Autodesk Fusion 360 part; units mm, degrees
note: some values were not read from the file. Chosen so that the rebuilt part matches the saved one: which face or edge a step refers to. Set by a fixed rule: which sketch regions a step uses.
(part 5 of 7)
  arc A238 (-20.6449, 76.0422) -> (-22.1292, 75.6235) centre (0, 0) ccw
  arc A239 (-20.6449, 76.0422) -> (-20.3501, 76.41) centre (-20.7497, 76.4282) ccw
  spline S239 degree 3 poles (-20.3133, 77.0419) (-20.3288, 76.8232) (-20.341, 76.6126) (-20.3501, 76.41) knots 0 0 0 0 1 1 1 1
  spline S240 degree 3 poles (-19.9812, 79.7947) (-20.1522, 78.771) (-20.2559, 77.8517) (-20.3133, 77.0419) knots 0 0 0 0 1 1 1 1
  arc A240 (-18.4227, 80.1689) -> (-19.9812, 79.7947) centre (0, 0) ccw
  spline S241 degree 3 poles (-16.877, 77.8669) (-17.2958, 78.5624) (-17.8055, 79.3344) (-18.4227, 80.1689) knots 0 0 0 0 1 1 1 1
  spline S242 degree 3 poles (-16.5573, 77.3206) (-16.6574, 77.4969) (-16.7639, 77.6791) (-16.877, 77.8669) knots 0 0 0 0 1 1 1 1
  arc A241 (-16.5573, 77.3206) -> (-16.1277, 77.1267) centre (-16.2095, 77.5182) ccw
  arc A242 (-14.6151, 77.4275) -> (-16.1277, 77.1267) centre (0, 0) ccw
  arc A243 (-14.6151, 77.4275) -> (-14.2923, 77.7712) centre (-14.6893, 77.8206) ccw
  spline S243 degree 3 poles (-14.2061, 78.3982) (-14.2387, 78.1814) (-14.2673, 77.9723) (-14.2923, 77.7712) knots 0 0 0 0 1 1 1 1
  spline S244 degree 3 poles (-13.659, 81.1164) (-13.9098, 80.1093) (-14.0853, 79.201) (-14.2061, 78.3982) knots 0 0 0 0 1 1 1 1
  arc A244 (-12.0759, 81.3672) -> (-13.659, 81.1164) centre (0, 0) ccw
  spline S245 degree 3 poles (-10.7156, 78.951) (-11.0785, 79.6772) (-11.5261, 80.4868) (-12.0759, 81.3672) knots 0 0 0 0 1 1 1 1
  spline S246 degree 3 poles (-10.4398, 78.3813) (-10.5258, 78.5649) (-10.6176, 78.7549) (-10.7156, 78.951) knots 0 0 0 0 1 1 1 1
  arc A245 (-10.4398, 78.3813) -> (-10.0267, 78.1543) centre (-10.0776, 78.551) ccw
  arc A246 (-8.4951, 78.3355) -> (-10.0267, 78.1543) centre (0, 0) ccw
  arc A247 (-8.4951, 78.3355) -> (-8.1464, 78.6528) centre (-8.5383, 78.7332) ccw
  spline S247 degree 3 poles (-8.0112, 79.2711) (-8.0608, 79.0575) (-8.1057, 78.8514) (-8.1464, 78.6528) knots 0 0 0 0 1 1 1 1
  spline S248 degree 3 poles (-7.2526, 81.938) (-7.5816, 80.9537) (-7.8278, 80.0619) (-8.0112, 79.2711) knots 0 0 0 0 1 1 1 1
  arc A248 (-5.6547, 82.0638) -> (-7.2526, 81.938) centre (0, 0) ccw
  spline S249 degree 3 poles (-4.4881, 79.5484) (-4.793, 80.3008) (-5.1757, 81.1431) (-5.6547, 82.0638) knots 0 0 0 0 1 1 1 1
  spline S250 degree 3 poles (-4.2579, 78.9588) (-4.3292, 79.1486) (-4.4058, 79.3452) (-4.4881, 79.5484) knots 0 0 0 0 1 1 1 1
  arc A249 (-4.2579, 78.9588) -> (-3.8638, 78.7) centre (-3.8835, 79.0995) ccw
  arc A250 (-2.3228, 78.7606) -> (-3.8638, 78.7) centre (0, 0) ccw
  arc A251 (-2.3228, 78.7606) -> (-1.9503, 79.0495) centre (-2.3346, 79.1604) ccw
  spline S251 degree 3 poles (-1.767, 79.6553) (-1.8331, 79.4462) (-1.8941, 79.2443) (-1.9503, 79.0495) knots 0 0 0 0 1 1 1 1
  spline S252 degree 3 poles (-0.8014, 82.2545) (-1.2067, 81.299) (-1.5221, 80.4293) (-1.767, 79.6553) knots 0 0 0 0 1 1 1 1
  arc A252 (0.8014, 82.2545) -> (-0.8014, 82.2545) centre (0, 0) ccw
  spline S253 degree 3 poles (1.767, 79.6553) (1.5221, 80.4293) (1.2067, 81.299) (0.8014, 82.2545) knots 0 0 0 0 1 1 1 1
  spline S254 degree 3 poles (1.9503, 79.0495) (1.8941, 79.2443) (1.8331, 79.4462) (1.767, 79.6553) knots 0 0 0 0 1 1 1 1
  arc A253 (1.9503, 79.0495) -> (2.3228, 78.7606) centre (2.3346, 79.1604) ccw
  arc A254 (3.8638, 78.7) -> (2.3228, 78.7606) centre (0, 0) ccw
  arc A255 (3.8638, 78.7) -> (4.2579, 78.9588) centre (3.8835, 79.0995) ccw
  spline S255 degree 3 poles (4.4881, 79.5484) (4.4058, 79.3452) (4.3292, 79.1486) (4.2579, 78.9588) knots 0 0 0 0 1 1 1 1
  spline S256 degree 3 poles (5.6547, 82.0638) (5.1757, 81.1431) (4.793, 80.3008) (4.4881, 79.5484) knots 0 0 0 0 1 1 1 1
  arc A256 (7.2526, 81.938) -> (5.6547, 82.0638) centre (0, 0) ccw
  spline S257 degree 3 poles (8.0112, 79.2711) (7.8278, 80.0619) (7.5816, 80.9537) (7.2526, 81.938) knots 0 0 0 0 1 1 1 1
  spline S258 degree 3 poles (8.1464, 78.6528) (8.1057, 78.8514) (8.0608, 79.0575) (8.0112, 79.2711) knots 0 0 0 0 1 1 1 1
  arc A257 (8.1464, 78.6528) -> (8.4951, 78.3355) centre (8.5383, 78.7332) ccw
  arc A258 (10.0267, 78.1543) -> (8.4951, 78.3355) centre (0, 0) ccw
  arc A259 (10.0267, 78.1543) -> (10.4398, 78.3813) centre (10.0776, 78.551) ccw
  spline S259 degree 3 poles (10.7156, 78.951) (10.6176, 78.7549) (10.5258, 78.5649) (10.4398, 78.3813) knots 0 0 0 0 1 1 1 1
  spline S260 degree 3 poles (12.0759, 81.3672) (11.5261, 80.4868) (11.0785, 79.6772) (10.7156, 78.951) knots 0 0 0 0 1 1 1 1
  arc A260 (13.659, 81.1164) -> (12.0759, 81.3672) centre (0, 0) ccw
  spline S261 degree 3 poles (14.2061, 78.3982) (14.0853, 79.201) (13.9098, 80.1093) (13.659, 81.1164) knots 0 0 0 0 1 1 1 1
  spline S262 degree 3 poles (14.2923, 77.7712) (14.2673, 77.9723) (14.2387, 78.1814) (14.2061, 78.3982) knots 0 0 0 0 1 1 1 1
  arc A261 (14.2923, 77.7712) -> (14.6151, 77.4275) centre (14.6893, 77.8206) ccw
  arc A262 (16.1277, 77.1267) -> (14.6151, 77.4275) centre (0, 0) ccw
  arc A263 (16.1277, 77.1267) -> (16.5573, 77.3206) centre (16.2095, 77.5182) ccw
  spline S263 degree 3 poles (16.877, 77.8669) (16.7639, 77.6791) (16.6574, 77.4969) (16.5573, 77.3206) knots 0 0 0 0 1 1 1 1
  spline S264 degree 3 poles (18.4227, 80.1689) (17.8055, 79.3344) (17.2958, 78.5624) (16.877, 77.8669) knots 0 0 0 0 1 1 1 1
  arc A264 (19.9812, 79.7947) -> (18.4227, 80.1689) centre (0, 0) ccw
  spline S265 degree 3 poles (20.3133, 77.0419) (20.2559, 77.8517) (20.1522, 78.771) (19.9812, 79.7947) knots 0 0 0 0 1 1 1 1
  spline S266 degree 3 poles (20.3501, 76.41) (20.341, 76.6126) (20.3288, 76.8232) (20.3133, 77.0419) knots 0 0 0 0 1 1 1 1
  arc A265 (20.3501, 76.41) -> (20.6449, 76.0422) centre (20.7497, 76.4282) ccw
  arc A266 (22.1292, 75.6235) -> (20.6449, 76.0422) centre (0, 0) ccw
  arc A267 (22.1292, 75.6235) -> (22.5728, 75.7832) centre (22.2416, 76.0074) ccw
  spline S267 degree 3 poles (22.9343, 76.3027) (22.8068, 76.1243) (22.6864, 75.9511) (22.5728, 75.7832) knots 0 0 0 0 1 1 1 1
  spline S268 degree 3 poles (24.6558, 78.4763) (23.9752, 77.6928) (23.4064, 76.9632) (22.9343, 76.3027) knots 0 0 0 0 1 1 1 1
  arc A268 (26.1802, 77.981) -> (24.6558, 78.4763) centre (0, 0) ccw
  spline S269 degree 3 poles (26.2953, 75.2107) (26.3016, 76.0225) (26.2704, 76.9471) (26.1802, 77.981) knots 0 0 0 0 1 1 1 1
  spline S270 degree 3 poles (26.2825, 74.5778) (26.2892, 74.7805) (26.2937, 74.9914) (26.2953, 75.2107) knots 0 0 0 0 1 1 1 1
  arc A269 (26.2825, 74.5778) -> (26.5475, 74.188) centre (26.6822, 74.5646) ccw
  arc A270 (27.9944, 73.6542) -> (26.5475, 74.188) centre (0, 0) ccw
  arc A271 (27.9944, 73.6542) -> (28.4491, 73.7785) centre (28.1365, 74.0281) ccw
  spline S271 degree 3 poles (28.8503, 74.2681) (28.7092, 74.1003) (28.5755, 73.937) (28.4491, 73.7785) knots 0 0 0 0 1 1 1 1
  spline S272 degree 3 poles (30.737, 76.2999) (29.997, 75.5723) (29.3727, 74.8895) (28.8503, 74.2681) knots 0 0 0 0 1 1 1 1
  arc A272 (32.2178, 75.6865) -> (30.737, 76.2999) centre (0, 0) ccw
  spline S273 degree 3 poles (32.1152, 72.9157) (32.1852, 73.7245) (32.2266, 74.6487) (32.2178, 75.6865) knots 0 0 0 0 1 1 1 1
  spline S274 degree 3 poles (32.0528, 72.2858) (32.0754, 72.4873) (32.0964, 72.6972) (32.1152, 72.9157) knots 0 0 0 0 1 1 1 1
  arc A273 (32.0528, 72.2858) -> (32.2864, 71.8764) centre (32.4503, 72.2413) ccw
  arc A274 (33.6869, 71.2307) -> (32.2864, 71.8764) centre (0, 0) ccw
  arc A275 (33.6869, 71.2307) -> (34.15, 71.319) centre (33.8579, 71.5923) ccw
  spline S275 degree 3 poles (34.5883, 71.7756) (34.4345, 71.6193) (34.2885, 71.4671) (34.15, 71.319) knots 0 0 0 0 1 1 1 1
  spline S276 degree 3 poles (36.6287, 73.6531) (35.8338, 72.9858) (35.1579, 72.3541) (34.5883, 71.7756) knots 0 0 0 0 1 1 1 1
  arc A276 (38.0568, 72.9254) -> (36.6287, 73.6531) centre (0, 0) ccw
  spline S277 degree 3 poles (37.7371, 70.1712) (37.8704, 70.972) (37.9841, 71.8901) (38.0568, 72.9254) knots 0 0 0 0 1 1 1 1
  spline S278 degree 3 poles (37.6254, 69.5482) (37.6638, 69.7473) (37.7012, 69.9549) (37.7371, 70.1712) knots 0 0 0 0 1 1 1 1
  arc A277 (37.6254, 69.5482) -> (37.8262, 69.1217) centre (38.0182, 69.4726) ccw
  arc A278 (39.1718, 68.3681) -> (37.8262, 69.1217) centre (0, 0) ccw
  arc A279 (39.1718, 68.3681) -> (39.6403, 68.4198) centre (39.3706, 68.7152) ccw
  spline S279 degree 3 poles (40.1132, 68.8406) (39.9475, 68.6969) (39.79, 68.5565) (39.6403, 68.4198) knots 0 0 0 0 1 1 1 1
  spline S280 degree 3 poles (42.2945, 70.5522) (41.4498, 69.9493) (40.7264, 69.3726) (40.1132, 68.8406) knots 0 0 0 0 1 1 1 1
  arc A280 (43.6612, 69.7147) -> (42.2945, 70.5522) centre (0, 0) ccw
  spline S281 degree 3 poles (43.1264, 66.9941) (43.322, 67.7819) (43.5075, 68.6883) (43.6612, 69.7147) knots 0 0 0 0 1 1 1 1
  spline S282 degree 3 poles (42.9661, 66.3817) (43.02, 66.5772) (43.0736, 66.7812) (43.1264, 66.9941) knots 0 0 0 0 1 1 1 1
  arc A281 (42.9661, 66.3817) -> (43.1328, 65.9408) centre (43.3518, 66.2755) ccw
  arc A282 (44.4151, 65.084) -> (43.1328, 65.9408) centre (0, 0) ccw
  arc A283 (44.4151, 65.084) -> (44.8863, 65.0987) centre (44.6406, 65.4144) ccw
  spline S283 degree 3 poles (45.3907, 65.4811) (45.2143, 65.3508) (45.0463, 65.2233) (44.8863, 65.0987) knots 0 0 0 0 1 1 1 1
  spline S284 degree 3 poles (47.6996, 67.0163) (46.8101, 66.4815) (46.0437, 65.9633) (45.3907, 65.4811) knots 0 0 0 0 1 1 1 1
  arc A284 (48.9963, 66.0742) -> (47.6996, 67.0163) centre (0, 0) ccw
  spline S285 degree 3 poles (48.2497, 63.4039) (48.5066, 64.174) (48.7626, 65.063) (48.9963, 66.0742) knots 0 0 0 0 1 1 1 1
  spline S286 degree 3 poles (48.0419, 62.806) (48.111, 62.9966) (48.1804, 63.1959) (48.2497, 63.4039) knots 0 0 0 0 1 1 1 1
  arc A285 (48.0419, 62.806) -> (48.1735, 62.3533) centre (48.418, 62.6699) ccw
  arc A286 (49.3846, 61.3986) -> (48.1735, 62.3533) centre (0, 0) ccw
  arc A287 (49.3846, 61.3986) -> (49.8555, 61.3763) centre (49.6353, 61.7102) ccw
  spline S287 degree 3 poles (50.3883, 61.7179) (50.2023, 61.6019) (50.0247, 61.4879) (49.8555, 61.3763) knots 0 0 0 0 1 1 1 1
  spline S288 degree 3 poles (52.8106, 63.0673) (51.8819, 62.6039) (51.0772, 62.1475) (50.3883, 61.7179) knots 0 0 0 0 1 1 1 1
  arc A288 (54.0294, 62.0263) -> (52.8106, 63.0673) centre (0, 0) ccw
  spline S289 degree 3 poles (53.0756, 59.4228) (53.3921, 60.1704) (53.717, 61.0366) (54.0294, 62.0263) knots 0 0 0 0 1 1 1 1
  spline S290 degree 3 poles (52.8215, 58.8431) (52.9053, 59.0277) (52.9901, 59.2209) (53.0756, 59.4228) knots 0 0 0 0 1 1 1 1
  arc A289 (52.8215, 58.8431) -> (52.9172, 58.3815) centre (53.1858, 58.6778) ccw
  arc A290 (54.0497, 57.3346) -> (52.9172, 58.3815) centre (0, 0) ccw
  arc A291 (54.0497, 57.3346) -> (54.5174, 57.2755) centre (54.324, 57.6257) ccw
  spline S291 degree 3 poles (55.0753, 57.5742) (54.8807, 57.4732) (54.6948, 57.3735) (54.5174, 57.2755) knots 0 0 0 0 1 1 1 1
  spline S292 degree 3 poles (57.596, 58.7294) (56.6338, 58.3403) (55.7958, 57.9484) (55.0753, 57.5742) knots 0 0 0 0 1 1 1 1
  arc A292 (58.7294, 57.596) -> (57.596, 58.7294) centre (0, 0) ccw
  spline S293 degree 3 poles (57.5742, 55.0753) (57.9484, 55.7958) (58.3403, 56.6338) (58.7294, 57.596) knots 0 0 0 0 1 1 1 1
  spline S294 degree 3 poles (57.2755, 54.5174) (57.3735, 54.6948) (57.4732, 54.8807) (57.5742, 55.0753) knots 0 0 0 0 1 1 1 1
  arc A293 (57.2755, 54.5174) -> (57.3346, 54.0497) centre (57.6257, 54.324) ccw
  arc A294 (58.3815, 52.9172) -> (57.3346, 54.0497) centre (0, 0) ccw
  arc A295 (58.3815, 52.9172) -> (58.8431, 52.8215) centre (58.6778, 53.1858) ccw
  spline S295 degree 3 poles (59.4228, 53.0756) (59.2209, 52.9901) (59.0277, 52.9053) (58.8431, 52.8215) knots 0 0 0 0 1 1 1 1
  spline S296 degree 3 poles (62.0263, 54.0294) (61.0366, 53.717) (60.1704, 53.3921) (59.4228, 53.0756) knots 0 0 0 0 1 1 1 1
  arc A296 (63.0673, 52.8106) -> (62.0263, 54.0294) centre (0, 0) ccw
  spline S297 degree 3 poles (61.7179, 50.3883) (62.1475, 51.0772) (62.6039, 51.8819) (63.0673, 52.8106) knots 0 0 0 0 1 1 1 1
  spline S298 degree 3 poles (61.3763, 49.8555) (61.4879, 50.0247) (61.6019, 50.2023) (61.7179, 50.3883) knots 0 0 0 0 1 1 1 1
  arc A297 (61.3763, 49.8555) -> (61.3986, 49.3846) centre (61.7102, 49.6353) ccw
  arc A298 (62.3533, 48.1735) -> (61.3986, 49.3846) centre (0, 0) ccw
  arc A299 (62.3533, 48.1735) -> (62.806, 48.0419) centre (62.6699, 48.418) ccw
  spline S299 degree 3 poles (63.4039, 48.2497) (63.1959, 48.1804) (62.9966, 48.111) (62.806, 48.0419) knots 0 0 0 0 1 1 1 1
  spline S300 degree 3 poles (66.0742, 48.9963) (65.063, 48.7626) (64.174, 48.5066) (63.4039, 48.2497) knots 0 0 0 0 1 1 1 1
  arc A300 (67.0163, 47.6996) -> (66.0742, 48.9963) centre (0, 0) ccw
  spline S301 degree 3 poles (65.4811, 45.3907) (65.9633, 46.0437) (66.4815, 46.8101) (67.0163, 47.6996) knots 0 0 0 0 1 1 1 1
  spline S302 degree 3 poles (65.0987, 44.8863) (65.2233, 45.0463) (65.3508, 45.2143) (65.4811, 45.3907) knots 0 0 0 0 1 1 1 1
  arc A301 (65.0987, 44.8863) -> (65.084, 44.4151) centre (65.4144, 44.6406) ccw
  arc A302 (65.9408, 43.1328) -> (65.084, 44.4151) centre (0, 0) ccw
  arc A303 (65.9408, 43.1328) -> (66.3817, 42.9661) centre (66.2755, 43.3518) ccw
  spline S303 degree 3 poles (66.9941, 43.1264) (66.7812, 43.0736) (66.5772, 43.02) (66.3817, 42.9661) knots 0 0 0 0 1 1 1 1
  spline S304 degree 3 poles (69.7147, 43.6612) (68.6883, 43.5075) (67.7819, 43.322) (66.9941, 43.1264) knots 0 0 0 0 1 1 1 1
  arc A304 (70.5522, 42.2945) -> (69.7147, 43.6612) centre (0, 0) ccw
  spline S305 degree 3 poles (68.8406, 40.1132) (69.3726, 40.7264) (69.9493, 41.4498) (70.5522, 42.2945) knots 0 0 0 0 1 1 1 1
  spline S306 degree 3 poles (68.4198, 39.6403) (68.5565, 39.79) (68.6969, 39.9475) (68.8406, 40.1132) knots 0 0 0 0 1 1 1 1
  arc A305 (68.4198, 39.6403) -> (68.3681, 39.1718) centre (68.7152, 39.3706) ccw
  arc A306 (69.1217, 37.8262) -> (68.3681, 39.1718) centre (0, 0) ccw
  arc A307 (69.1217, 37.8262) -> (69.5482, 37.6254) centre (69.4726, 38.0182) ccw
  spline S307 degree 3 poles (70.1712, 37.7371) (69.9549, 37.7012) (69.7473, 37.6638) (69.5482, 37.6254) knots 0 0 0 0 1 1 1 1
  spline S308 degree 3 poles (72.9254, 38.0568) (71.8901, 37.9841) (70.972, 37.8704) (70.1712, 37.7371) knots 0 0 0 0 1 1 1 1
  arc A308 (73.6531, 36.6287) -> (72.9254, 38.0568) centre (0, 0) ccw
  spline S309 degree 3 poles (71.7756, 34.5883) (72.3541, 35.1579) (72.9858, 35.8338) (73.6531, 36.6287) knots 0 0 0 0 1 1 1 1
  spline S310 degree 3 poles (71.319, 34.15) (71.4671, 34.2885) (71.6193, 34.4345) (71.7756, 34.5883) knots 0 0 0 0 1 1 1 1
  arc A309 (71.319, 34.15) -> (71.2307, 33.6869) centre (71.5923, 33.8579) ccw
  arc A310 (71.8764, 32.2864) -> (71.2307, 33.6869) centre (0, 0) ccw
  arc A311 (71.8764, 32.2864) -> (72.2858, 32.0528) centre (72.2413, 32.4503) ccw
  spline S311 degree 3 poles (72.9157, 32.1152) (72.6972, 32.0964) (72.4873, 32.0754) (72.2858, 32.0528) knots 0 0 0 0 1 1 1 1
  spline S312 degree 3 poles (75.6865, 32.2178) (74.6487, 32.2266) (73.7245, 32.1852) (72.9157, 32.1152) knots 0 0 0 0 1 1 1 1
  arc A312 (76.2999, 30.737) -> (75.6865, 32.2178) centre (0, 0) ccw
  spline S313 degree 3 poles (74.2681, 28.8503) (74.8895, 29.3727) (75.5723, 29.997) (76.2999, 30.737) knots 0 0 0 0 1 1 1 1
  spline S314 degree 3 poles (73.7785, 28.4491) (73.937, 28.5755) (74.1003, 28.7092) (74.2681, 28.8503) knots 0 0 0 0 1 1 1 1
  arc A313 (73.7785, 28.4491) -> (73.6542, 27.9944) centre (74.0281, 28.1365) ccw
  arc A314 (74.188, 26.5475) -> (73.6542, 27.9944) centre (0, 0) ccw
  arc A315 (74.188, 26.5475) -> (74.5778, 26.2825) centre (74.5646, 26.6822) ccw
  spline S315 degree 3 poles (75.2107, 26.2953) (74.9914, 26.2937) (74.7805, 26.2892) (74.5778, 26.2825) knots 0 0 0 0 1 1 1 1
  spline S316 degree 3 poles (77.981, 26.1802) (76.9471, 26.2704) (76.0225, 26.3016) (75.2107, 26.2953) knots 0 0 0 0 1 1 1 1
  arc A316 (78.4763, 24.6558) -> (77.981, 26.1802) centre (0, 0) ccw
  spline S317 degree 3 poles (76.3027, 22.9343) (76.9632, 23.4064) (77.6928, 23.9752) (78.4763, 24.6558) knots 0 0 0 0 1 1 1 1
  spline S318 degree 3 poles (75.7832, 22.5728) (75.9511, 22.6864) (76.1243, 22.8068) (76.3027, 22.9343) knots 0 0 0 0 1 1 1 1
  arc A317 (75.7832, 22.5728) -> (75.6235, 22.1292) centre (76.0074, 22.2416) ccw
  arc A318 (76.0422, 20.6449) -> (75.6235, 22.1292) centre (0, 0) ccw
  arc A319 (76.0422, 20.6449) -> (76.41, 20.3501) centre (76.4282, 20.7497) ccw
  spline S319 degree 3 poles (77.0419, 20.3133) (76.8232, 20.3288) (76.6126, 20.341) (76.41, 20.3501) knots 0 0 0 0 1 1 1 1
  circle A320 centre (0, 0) radius 92.5
  circle A321 centre (-0.23, 87.5037) radius 5
  circle A322 centre (-75.6654, -43.951) radius 5
  circle A323 centre (75.8954, -43.5527) radius 5
  dimension "d70" = 10
  dimension "d72" = 360
  measures "d70" diameter of A321
extrude "Extrude2" add sketch "Sketch15" along normal blind 12 contours A320 A321 | A320 A323 | A320 A322 picked at (-0.0821, 85.8471) picked at (74.5605, -42.5553) picked at (-74.1888, -43.1909) bodies 3 in component "Internal Gear (80 teeth)"
sketch "Sketch16" plane through (0, 20, 0) normal (0, 1, 0) x (-1, 0, 0)
  circle A0 centre (-41.6795, 43.1604) radius 5.25
  line L0 (-40.2809, 27.3166) -> (-53.3344, 40.8338)
  line L1 (-25.8942, 41.2097) -> (-38.9476, 54.727)
  arc A1 (-40.9244, 55.6376) -> (-54.1754, 42.8412) centre (-41.6795, 43.1604) ccw
  circle A2 centre (-16.5382, -57.6757) radius 5.25
  arc A3 (-27.7213, -63.2604) -> (-10.0139, -68.3379) centre (-16.5382, -57.6757) ccw
  line L2 (-22.7416, -43.0299) -> (-27.9212, -61.0931)
  line L3 (-3.5164, -48.5426) -> (-8.6959, -66.6059)
  circle A4 centre (58.2177, 14.5153) radius 5.25
  arc A5 (68.6458, 7.6228) -> (64.1893, 25.4967) centre (58.2177, 14.5153) ccw
  line L4 (48.6358, 1.8201) -> (66.8688, 6.3661)
  line L5 (43.7973, 21.226) -> (62.0304, 25.772)
  arc A6 (-22.7416, -43.0299) -> (-40.2809, 27.3166) centre (-92.4331, -23.0462) ccw
  arc A7 (-25.8942, 41.2097) -> (43.7973, 21.226) centre (26.258, 91.5725) ccw
  arc A8 (48.6358, 1.8201) -> (-3.5164, -48.5426) centre (66.1751, -68.5263) ccw
  arc A9 (64.1893, 25.4967) -> (62.0304, 25.772) centre (62.7561, 22.8612) ccw
  arc A10 (66.8688, 6.3661) -> (68.6458, 7.6228) centre (66.143, 9.277) ccw
  arc A11 (-54.1754, 42.8412) -> (-53.3344, 40.8338) centre (-51.1764, 42.9178) ccw
  arc A12 (-38.9476, 54.727) -> (-40.9244, 55.6376) centre (-41.1056, 52.643) ccw
  arc A13 (-27.9212, -61.0931) -> (-27.7213, -63.2604) centre (-25.0374, -61.9201) ccw
  arc A14 (-10.0139, -68.3379) -> (-8.6959, -66.6059) centre (-11.5797, -65.779) ccw
  dimension "d82" = 72.5
  dimension "d83" = 3
  dimension "d84" = 3
  measures "d82" radius of A6
  measures "d83" radius of A9
  measures "d84" radius of A10
extrude "Extrude1'''''" add sketch "Sketch16" against normal blind 8 separate body makes body 6 in component "Component''"
sketch "Sketch17" plane through (0, 20, 0) normal (0, 1, 0) x (-1, 0, 0)
  circle A0 centre (58.2177, 14.5153) radius 5.25
  circle A1 centre (-41.6795, 43.1604) radius 5.25
  circle A2 centre (-16.5382, -57.6757) radius 5.25
  line L0 (-22.7416, -43.0299) -> (-27.9212, -61.0931)
  arc A3 (-27.9212, -61.0931) -> (-27.7213, -63.2604) centre (-25.0374, -61.9201) ccw
  arc A4 (-27.7213, -63.2604) -> (-10.0139, -68.3379) centre (-16.5382, -57.6757) ccw
  arc A5 (-10.0139, -68.3379) -> (-8.6959, -66.6059) centre (-11.5797, -65.779) ccw
  line L1 (-8.6959, -66.6059) -> (-3.5164, -48.5426)
  arc A6 (48.6358, 1.8201) -> (-3.5164, -48.5426) centre (66.1751, -68.5263) ccw
  line L2 (48.6358, 1.8201) -> (66.8688, 6.3661)
  arc A7 (66.8688, 6.3661) -> (68.6458, 7.6228) centre (66.143, 9.277) ccw
  arc A8 (68.6458, 7.6228) -> (64.1893, 25.4967) centre (58.2177, 14.5153) ccw
  arc A9 (64.1893, 25.4967) -> (62.0304, 25.772) centre (62.7561, 22.8612) ccw
  line L3 (62.0304, 25.772) -> (43.7973, 21.226)
  arc A10 (-25.8942, 41.2097) -> (43.7973, 21.226) centre (26.258, 91.5725) ccw
  line L4 (-25.8942, 41.2097) -> (-38.9476, 54.727)
  arc A11 (-38.9476, 54.727) -> (-40.9244, 55.6376) centre (-41.1056, 52.643) ccw
  arc A12 (-40.9244, 55.6376) -> (-54.1754, 42.8412) centre (-41.6795, 43.1604) ccw
  arc A13 (-54.1754, 42.8412) -> (-53.3344, 40.8338) centre (-51.1764, 42.9178) ccw
  line L5 (-53.3344, 40.8338) -> (-40.2809, 27.3166)
  arc A14 (-22.7416, -43.0299) -> (-40.2809, 27.3166) centre (-92.4331, -23.0462) ccw
  circle A15 centre (0, 0) radius 3.85
  dimension "d87" = 7.7
  measures "d87" diameter of A15
extrude "Extrude2'" cut sketch "Sketch17" against normal blind 10 contours A15 bodies 6 in component "Component''"
sketch "Sketch18" plane through (0, 0, 0) normal (0, 1, 0) x (1, 0, 0)
  circle A0 centre (-0.103, 0.0004) radius 92.4999
extrude "Extrude1''''''" add sketch "Sketch18" against normal blind 8 from surface at -12 separate body makes body 7 in component "Component'''"
sketch "Sketch19" plane through (0, -20, 0) normal (0, -1, 0) x (1, 0, 0)
  circle A0 centre (-0.103, -0.0004) radius 92.4999
  arc A1 (-19.5205, 69.5982) -> (-70.2173, 17.1604) centre (0, 0) ccw
  arc A2 (-13.5027, 48.1423) -> (-19.5205, 69.5982) centre (-16.5116, 58.8702) ccw
  arc A3 (-13.5027, 48.1423) -> (-48.5706, 11.8702) centre (0, 0) ccw
  arc A4 (-70.2173, 17.1604) -> (-48.5706, 11.8702) centre (-59.3939, 14.5153) ccw
  arc A5 (-16.5116, 58.8702) -> (-59.3939, 14.5153) centre (0, 0) ccw construction
  arc A6 (20.2473, -69.3902) -> (14.0054, -47.9984) centre (17.1263, -58.6943) ccw
  arc A7 (-34.9411, -35.7648) -> (14.0054, -47.9984) centre (0, 0) ccw
  arc A8 (-34.9411, -35.7648) -> (-50.5135, -51.7043) centre (-42.7273, -43.7345) ccw
  arc A9 (-50.5135, -51.7043) -> (20.2473, -69.3902) centre (0, 0) ccw
  arc A10 (49.97, 52.2298) -> (34.5652, 36.1282) centre (42.2676, 44.179) ccw
  arc A11 (48.4438, -12.3775) -> (34.5652, 36.1282) centre (0, 0) ccw
  arc A12 (48.4438, -12.3775) -> (70.034, -17.8939) centre (59.2389, -15.1357) ccw
  arc A13 (70.034, -17.8939) -> (49.97, 52.2298) centre (0, 0) ccw
  dimension "d94" = 360
extrude "Extrude2''" cut sketch "Sketch19" against normal blind 8 contours A1 A2 A3 A4 | A6 A7 A8 A9 | A10 A11 A12 A13 bodies 7 in component "Component'''"
sketch "Sketch20" plane through (0, -20, 0) normal (0, -1, 0) x (1, 0, 0)
  arc A0 (70.034, -17.8939) -> (49.97, 52.2298) centre (0, 0) ccw
  arc A1 (48.4438, -12.3775) -> (70.034, -17.8939) centre (59.2389, -15.1357) ccw
  arc A2 (48.4438, -12.3775) -> (34.5652, 36.1282) centre (0, 0) ccw
  arc A3 (49.97, 52.2298) -> (34.5652, 36.1282) centre (42.2676, 44.179) ccw
  arc A4 (-19.5205, 69.5982) -> (-70.2173, 17.1604) centre (0, 0) ccw
  arc A5 (-13.5027, 48.1423) -> (-19.5205, 69.5982) centre (-16.5116, 58.8702) ccw
  arc A6 (-13.5027, 48.1423) -> (-48.5706, 11.8702) centre (0, 0) ccw
  arc A7 (-70.2173, 17.1604) -> (-48.5706, 11.8702) centre (-59.3939, 14.5153) ccw
  arc A8 (-50.5135, -51.7043) -> (20.2473, -69.3902) centre (0, 0) ccw
  arc A9 (-34.9411, -35.7648) -> (-50.5135, -51.7043) centre (-42.7273, -43.7345) ccw
  arc A10 (-34.9411, -35.7648) -> (14.0054, -47.9984) centre (0, 0) ccw
  arc A11 (20.2473, -69.3902) -> (14.0054, -47.9984) centre (17.1263, -58.6943) ccw
  circle A12 centre (-0.103, -0.0004) radius 92.4999
  circle A13 centre (-0.103, -0.0004) radius 4.35
  dimension "d97" = 8.7
  measures "d97" diameter of A13
extrude "Extrude3" cut sketch "Sketch20" against normal blind 11 contours A13 bodies 7 in component "Component'''"
sketch "Sketch21" plane through (0, 0, 0) normal (0, -1, 0) x (1, 0, 0)
  circle A0 centre (0, 0) radius 3.85
  spline S0 degree 3 poles (-20.7021, -31.9674) (-20.8297, -32.1213) (-21.0408, -32.3546) (-21.3609, -32.6493) knots 0 0 0 0 1 1 1 1
  arc A1 (-20.1803, -31.8848) -> (-20.7021, -31.9674) centre (-20.3942, -32.2228) ccw
  arc A2 (-20.1803, -31.8848) -> (-19.2479, -32.4562) centre (0, 0) ccw
  arc A3 (-19.0846, -32.9586) -> (-19.2479, -32.4562) centre (-19.4519, -32.8002) ccw
  spline S1 degree 3 poles (-19.3931, -33.8552) (-19.2759, -33.4362) (-19.1638, -33.1422) (-19.0846, -32.9586) knots 0 0 0 0 1 1 1 1
  spline S2 degree 3 poles (-19.866, -37.3046) (-19.823, -35.7503) (-19.6037, -34.6096) (-19.3931, -33.8552) knots 0 0 0 0 1 1 1 1
  arc A4 (-19.866, -37.3046) -> (-18.5031, -37.999) centre (0, 0) ccw
  spline S3 degree 3 poles (-15.9905, -35.5889) (-16.477, -36.2028) (-17.271, -37.0506) (-18.5031, -37.999) knots 0 0 0 0 1 1 1 1
  spline S4 degree 3 poles (-15.4464, -34.8123) (-15.5484, -34.9843) (-15.7204, -35.2478) (-15.9905, -35.5889) knots 0 0 0 0 1 1 1 1
  arc A5 (-14.944, -34.6491) -> (-15.4464, -34.8123) centre (-15.1024, -35.0164) ccw
  arc A6 (-14.944, -34.6491) -> (-13.9336, -35.0676) centre (0, 0) ccw
  arc A7 (-13.6938, -35.5383) -> (-13.9336, -35.0676) centre (-14.0813, -35.4393) ccw
  spline S5 degree 3 poles (-13.8582, -36.4722) (-13.808, -36.0399) (-13.7432, -35.732) (-13.6938, -35.5383) knots 0 0 0 0 1 1 1 1
  spline S6 degree 3 poles (-13.7857, -39.953) (-13.9863, -38.4112) (-13.9482, -37.2502) (-13.8582, -36.4722) knots 0 0 0 0 1 1 1 1
  arc A8 (-13.7857, -39.953) -> (-12.331, -40.4257) centre (0, 0) ccw
  spline S7 degree 3 poles (-10.2263, -37.6523) (-10.6107, -38.3346) (-11.2623, -39.2962) (-12.331, -40.4257) knots 0 0 0 0 1 1 1 1
  spline S8 degree 3 poles (-9.8104, -36.8001) (-9.8842, -36.9859) (-10.0128, -37.273) (-10.2263, -37.6523) knots 0 0 0 0 1 1 1 1
  arc A9 (-9.3397, -36.5603) -> (-9.8104, -36.8001) centre (-9.4387, -36.9478) ccw
  arc A10 (-9.3397, -36.5603) -> (-8.2763, -36.8156) centre (0, 0) ccw
  arc A11 (-7.9658, -37.243) -> (-8.2763, -36.8156) centre (-8.364, -37.2058) ccw
  spline S9 degree 3 poles (-7.9821, -38.191) (-8.0001, -37.7562) (-7.9843, -37.442) (-7.9658, -37.243) knots 0 0 0 0 1 1 1 1
  spline S10 degree 3 poles (-7.3659, -41.6177) (-7.8053, -40.1262) (-7.9493, -38.9736) (-7.9821, -38.191) knots 0 0 0 0 1 1 1 1
  arc A12 (-7.3659, -41.6177) -> (-5.8552, -41.857) centre (0, 0) ccw
  spline S11 degree 3 poles (-4.2102, -38.7884) (-4.4833, -39.5225) (-4.9764, -40.5743) (-5.8552, -41.857) knots 0 0 0 0 1 1 1 1
  spline S12 degree 3 poles (-3.9328, -37.8817) (-3.9767, -38.0767) (-4.0588, -38.3805) (-4.2102, -38.7884) knots 0 0 0 0 1 1 1 1
  arc A13 (-3.5054, -37.5712) -> (-3.9328, -37.8817) centre (-3.5426, -37.9695) ccw
  arc A14 (-3.5054, -37.5712) -> (-2.4152, -37.657) centre (0, 0) ccw
  arc A15 (-2.0416, -38.0306) -> (-2.4152, -37.657) centre (-2.4408, -38.0562) ccw
  spline S13 degree 3 poles (-1.9094, -38.9695) (-1.9952, -38.5429) (-2.0288, -38.23) (-2.0416, -38.0306) knots 0 0 0 0 1 1 1 1
  spline S14 degree 3 poles (-0.7648, -42.2576) (-1.4321, -40.8532) (-1.7546, -39.7373) (-1.9094, -38.9695) knots 0 0 0 0 1 1 1 1
  arc A16 (-0.7648, -42.2576) -> (0.7648, -42.2576) centre (0, 0) ccw
  spline S15 degree 3 poles (1.9094, -38.9695) (1.7546, -39.7373) (1.4321, -40.8532) (0.7648, -42.2576) knots 0 0 0 0 1 1 1 1
  spline S16 degree 3 poles (2.0416, -38.0306) (2.0288, -38.23) (1.9952, -38.5429) (1.9094, -38.9695) knots 0 0 0 0 1 1 1 1
  arc A17 (2.4152, -37.657) -> (2.0416, -38.0306) centre (2.4408, -38.0562) ccw
  arc A18 (2.4152, -37.657) -> (3.5054, -37.5712) centre (0, 0) ccw
  arc A19 (3.9328, -37.8817) -> (3.5054, -37.5712) centre (3.5426, -37.9695) ccw
  spline S17 degree 3 poles (4.2102, -38.7884) (4.0588, -38.3805) (3.9767, -38.0767) (3.9328, -37.8817) knots 0 0 0 0 1 1 1 1
  spline S18 degree 3 poles (5.8552, -41.857) (4.9764, -40.5743) (4.4833, -39.5225) (4.2102, -38.7884) knots 0 0 0 0 1 1 1 1
  arc A20 (5.8552, -41.857) -> (7.3659, -41.6177) centre (0, 0) ccw
  spline S19 degree 3 poles (7.9821, -38.191) (7.9493, -38.9736) (7.8053, -40.1262) (7.3659, -41.6177) knots 0 0 0 0 1 1 1 1
  spline S20 degree 3 poles (7.9658, -37.243) (7.9843, -37.442) (8.0001, -37.7562) (7.9821, -38.191) knots 0 0 0 0 1 1 1 1
  arc A21 (8.2763, -36.8156) -> (7.9658, -37.243) centre (8.364, -37.2058) ccw
  arc A22 (8.2763, -36.8156) -> (9.3397, -36.5603) centre (0, 0) ccw
  arc A23 (9.8104, -36.8001) -> (9.3397, -36.5603) centre (9.4387, -36.9478) ccw
  spline S21 degree 3 poles (10.2263, -37.6523) (10.0128, -37.273) (9.8842, -36.9859) (9.8104, -36.8001) knots 0 0 0 0 1 1 1 1
  spline S22 degree 3 poles (12.331, -40.4257) (11.2623, -39.2962) (10.6107, -38.3346) (10.2263, -37.6523) knots 0 0 0 0 1 1 1 1
  arc A24 (12.331, -40.4257) -> (13.7857, -39.953) centre (0, 0) ccw
  spline S23 degree 3 poles (13.8582, -36.4722) (13.9482, -37.2502) (13.9863, -38.4112) (13.7857, -39.953) knots 0 0 0 0 1 1 1 1
  spline S24 degree 3 poles (13.6938, -35.5383) (13.7432, -35.732) (13.808, -36.0399) (13.8582, -36.4722) knots 0 0 0 0 1 1 1 1
  arc A25 (13.9336, -35.0676) -> (13.6938, -35.5383) centre (14.0813, -35.4393) ccw
  arc A26 (13.9336, -35.0676) -> (14.944, -34.6491) centre (0, 0) ccw
  arc A27 (15.4464, -34.8123) -> (14.944, -34.6491) centre (15.1024, -35.0164) ccw
  spline S25 degree 3 poles (15.9905, -35.5889) (15.7204, -35.2478) (15.5484, -34.9843) (15.4464, -34.8123) knots 0 0 0 0 1 1 1 1
  spline S26 degree 3 poles (18.5031, -37.999) (17.271, -37.0506) (16.477, -36.2028) (15.9905, -35.5889) knots 0 0 0 0 1 1 1 1
  arc A28 (18.5031, -37.999) -> (19.866, -37.3046) centre (0, 0) ccw
  spline S27 degree 3 poles (19.3931, -33.8552) (19.6037, -34.6096) (19.823, -35.7503) (19.866, -37.3046) knots 0 0 0 0 1 1 1 1
  spline S28 degree 3 poles (19.0846, -32.9586) (19.1638, -33.1422) (19.2759, -33.4362) (19.3931, -33.8552) knots 0 0 0 0 1 1 1 1
  arc A29 (19.2479, -32.4562) -> (19.0846, -32.9586) centre (19.4519, -32.8002) ccw
  arc A30 (19.2479, -32.4562) -> (20.1803, -31.8848) centre (0, 0) ccw
  arc A31 (20.7021, -31.9674) -> (20.1803, -31.8848) centre (20.3942, -32.2228) ccw
  spline S29 degree 3 poles (21.3609, -32.6493) (21.0408, -32.3546) (20.8297, -32.1213) (20.7021, -31.9674) knots 0 0 0 0 1 1 1 1
  spline S30 degree 3 poles (24.2197, -34.6367) (22.8543, -33.8927) (21.9375, -33.1795) (21.3609, -32.6493) knots 0 0 0 0 1 1 1 1
  arc A32 (24.2197, -34.6367) -> (25.4571, -33.7376) centre (0, 0) ccw
  spline S31 degree 3 poles (24.4505, -30.4047) (24.7765, -31.1168) (25.1715, -32.2092) (25.4571, -33.7376) knots 0 0 0 0 1 1 1 1
  spline S32 degree 3 poles (24.0055, -29.5673) (24.1124, -29.7363) (24.2691, -30.0091) (24.4505, -30.4047) knots 0 0 0 0 1 1 1 1
  arc A33 (24.0882, -29.0455) -> (24.0055, -29.5673) centre (24.3435, -29.3534) ccw
  arc A34 (24.0882, -29.0455) -> (24.9197, -28.3353) centre (0, 0) ccw
  arc A35 (25.448, -28.3353) -> (24.9197, -28.3353) centre (25.1839, -28.6357) ccw
  spline S33 degree 3 poles (26.2054, -28.9058) (25.8431, -28.6648) (25.5981, -28.4673) (25.448, -28.3353) knots 0 0 0 0 1 1 1 1
  spline S34 degree 3 poles (29.3399, -30.4214) (27.8749, -29.9002) (26.8578, -29.3392) (26.2054, -28.9058) knots 0 0 0 0 1 1 1 1
  arc A36 (29.3399, -30.4214) -> (30.4214, -29.3399) centre (0, 0) ccw
  spline S35 degree 3 poles (28.9058, -26.2054) (29.3392, -26.8578) (29.9002, -27.8749) (30.4214, -29.3399) knots 0 0 0 0 1 1 1 1
  spline S36 degree 3 poles (28.3353, -25.448) (28.4673, -25.5981) (28.6648, -25.8431) (28.9058, -26.2054) knots 0 0 0 0 1 1 1 1
  arc A37 (28.3353, -24.9197) -> (28.3353, -25.448) centre (28.6357, -25.1839) ccw
  arc A38 (28.3353, -24.9197) -> (29.0455, -24.0882) centre (0, 0) ccw
  arc A39 (29.5673, -24.0055) -> (29.0455, -24.0882) centre (29.3534, -24.3435) ccw
  spline S37 degree 3 poles (30.4047, -24.4505) (30.0091, -24.2691) (29.7363, -24.1124) (29.5673, -24.0055) knots 0 0 0 0 1 1 1 1
  spline S38 degree 3 poles (33.7376, -25.4571) (32.2092, -25.1715) (31.1168, -24.7765) (30.4047, -24.4505) knots 0 0 0 0 1 1 1 1
  arc A40 (33.7376, -25.4571) -> (34.6367, -24.2197) centre (0, 0) ccw
  spline S39 degree 3 poles (32.6493, -21.3609) (33.1795, -21.9375) (33.8927, -22.8543) (34.6367, -24.2197) knots 0 0 0 0 1 1 1 1
  spline S40 degree 3 poles (31.9674, -20.7021) (32.1213, -20.8297) (32.3546, -21.0408) (32.6493, -21.3609) knots 0 0 0 0 1 1 1 1
  arc A41 (31.8848, -20.1803) -> (31.9674, -20.7021) centre (32.2228, -20.3942) ccw
  arc A42 (31.8848, -20.1803) -> (32.4562, -19.2479) centre (0, 0) ccw
  arc A43 (32.9586, -19.0846) -> (32.4562, -19.2479) centre (32.8002, -19.4519) ccw
  spline S41 degree 3 poles (33.8552, -19.3931) (33.4362, -19.2759) (33.1422, -19.1638) (32.9586, -19.0846) knots 0 0 0 0 1 1 1 1
  spline S42 degree 3 poles (37.3046, -19.866) (35.7503, -19.823) (34.6096, -19.6037) (33.8552, -19.3931) knots 0 0 0 0 1 1 1 1
  arc A44 (37.3046, -19.866) -> (37.999, -18.5031) centre (0, 0) ccw
  spline S43 degree 3 poles (35.5889, -15.9905) (36.2028, -16.477) (37.0506, -17.271) (37.999, -18.5031) knots 0 0 0 0 1 1 1 1
  spline S44 degree 3 poles (34.8123, -15.4464) (34.9843, -15.5484) (35.2478, -15.7204) (35.5889, -15.9905) knots 0 0 0 0 1 1 1 1
  arc A45 (34.6491, -14.944) -> (34.8123, -15.4464) centre (35.0164, -15.1024) ccw
  arc A46 (34.6491, -14.944) -> (35.0676, -13.9336) centre (0, 0) ccw
  arc A47 (35.5383, -13.6938) -> (35.0676, -13.9336) centre (35.4393, -14.0813) ccw
  spline S45 degree 3 poles (36.4722, -13.8582) (36.0399, -13.808) (35.732, -13.7432) (35.5383, -13.6938) knots 0 0 0 0 1 1 1 1
  spline S46 degree 3 poles (39.953, -13.7857) (38.4112, -13.9863) (37.2502, -13.9482) (36.4722, -13.8582) knots 0 0 0 0 1 1 1 1
  arc A48 (39.953, -13.7857) -> (40.4257, -12.331) centre (0, 0) ccw
  spline S47 degree 3 poles (37.6523, -10.2263) (38.3346, -10.6107) (39.2962, -11.2623) (40.4257, -12.331) knots 0 0 0 0 1 1 1 1
  spline S48 degree 3 poles (36.8001, -9.8104) (36.9859, -9.8842) (37.273, -10.0128) (37.6523, -10.2263) knots 0 0 0 0 1 1 1 1
  arc A49 (36.5603, -9.3397) -> (36.8001, -9.8104) centre (36.9478, -9.4387) ccw
  arc A50 (36.5603, -9.3397) -> (36.8156, -8.2763) centre (0, 0) ccw
  arc A51 (37.243, -7.9658) -> (36.8156, -8.2763) centre (37.2058, -8.364) ccw
  spline S49 degree 3 poles (38.191, -7.9821) (37.7562, -8.0001) (37.442, -7.9843) (37.243, -7.9658) knots 0 0 0 0 1 1 1 1
  spline S50 degree 3 poles (41.6177, -7.3659) (40.1262, -7.8053) (38.9736, -7.9493) (38.191, -7.9821) knots 0 0 0 0 1 1 1 1
  arc A52 (41.6177, -7.3659) -> (41.857, -5.8552) centre (0, 0) ccw
  spline S51 degree 3 poles (38.7884, -4.2102) (39.5225, -4.4833) (40.5743, -4.9764) (41.857, -5.8552) knots 0 0 0 0 1 1 1 1
  spline S52 degree 3 poles (37.8817, -3.9328) (38.0767, -3.9767) (38.3805, -4.0588) (38.7884, -4.2102) knots 0 0 0 0 1 1 1 1
  arc A53 (37.5712, -3.5054) -> (37.8817, -3.9328) centre (37.9695, -3.5426) ccw
  arc A54 (37.5712, -3.5054) -> (37.657, -2.4152) centre (0, 0) ccw
  arc A55 (38.0306, -2.0416) -> (37.657, -2.4152) centre (38.0562, -2.4408) ccw
  spline S53 degree 3 poles (38.9695, -1.9094) (38.5429, -1.9952) (38.23, -2.0288) (38.0306, -2.0416) knots 0 0 0 0 1 1 1 1
  spline S54 degree 3 poles (42.2576, -0.7648) (40.8532, -1.4321) (39.7373, -1.7546) (38.9695, -1.9094) knots 0 0 0 0 1 1 1 1
  arc A56 (42.2576, -0.7648) -> (42.2576, 0.7648) centre (0, 0) ccw
  spline S55 degree 3 poles (38.9695, 1.9094) (39.7373, 1.7546) (40.8532, 1.4321) (42.2576, 0.7648) knots 0 0 0 0 1 1 1 1
  spline S56 degree 3 poles (38.0306, 2.0416) (38.23, 2.0288) (38.5429, 1.9952) (38.9695, 1.9094) knots 0 0 0 0 1 1 1 1
  arc A57 (37.657, 2.4152) -> (38.0306, 2.0416) centre (38.0562, 2.4408) ccw
  arc A58 (37.657, 2.4152) -> (37.5712, 3.5054) centre (0, 0) ccw
  arc A59 (37.8817, 3.9328) -> (37.5712, 3.5054) centre (37.9695, 3.5426) ccw
  spline S57 degree 3 poles (38.7884, 4.2102) (38.3805, 4.0588) (38.0767, 3.9767) (37.8817, 3.9328) knots 0 0 0 0 1 1 1 1
  spline S58 degree 3 poles (41.857, 5.8552) (40.5743, 4.9764) (39.5225, 4.4833) (38.7884, 4.2102) knots 0 0 0 0 1 1 1 1
  arc A60 (41.857, 5.8552) -> (41.6177, 7.3659) centre (0, 0) ccw
  spline S59 degree 3 poles (38.191, 7.9821) (38.9736, 7.9493) (40.1262, 7.8053) (41.6177, 7.3659) knots 0 0 0 0 1 1 1 1
  spline S60 degree 3 poles (37.243, 7.9658) (37.442, 7.9843) (37.7562, 8.0001) (38.191, 7.9821) knots 0 0 0 0 1 1 1 1
  arc A61 (36.8156, 8.2763) -> (37.243, 7.9658) centre (37.2058, 8.364) ccw
  arc A62 (36.8156, 8.2763) -> (36.5603, 9.3397) centre (0, 0) ccw
  arc A63 (36.8001, 9.8104) -> (36.5603, 9.3397) centre (36.9478, 9.4387) ccw
  spline S61 degree 3 poles (37.6523, 10.2263) (37.273, 10.0128) (36.9859, 9.8842) (36.8001, 9.8104) knots 0 0 0 0 1 1 1 1
  spline S62 degree 3 poles (40.4257, 12.331) (39.2962, 11.2623) (38.3346, 10.6107) (37.6523, 10.2263) knots 0 0 0 0 1 1 1 1
  arc A64 (40.4257, 12.331) -> (39.953, 13.7857) centre (0, 0) ccw
  spline S63 degree 3 poles (36.4722, 13.8582) (37.2502, 13.9482) (38.4112, 13.9863) (39.953, 13.7857) knots 0 0 0 0 1 1 1 1
  spline S64 degree 3 poles (35.5383, 13.6938) (35.732, 13.7432) (36.0399, 13.808) (36.4722, 13.8582) knots 0 0 0 0 1 1 1 1
  arc A65 (35.0676, 13.9336) -> (35.5383, 13.6938) centre (35.4393, 14.0813) ccw
  arc A66 (35.0676, 13.9336) -> (34.6491, 14.944) centre (0, 0) ccw
  arc A67 (34.8123, 15.4464) -> (34.6491, 14.944) centre (35.0164, 15.1024) ccw
  spline S65 degree 3 poles (35.5889, 15.9905) (35.2478, 15.7204) (34.9843, 15.5484) (34.8123, 15.4464) knots 0 0 0 0 1 1 1 1
  spline S66 degree 3 poles (37.999, 18.5031) (37.0506, 17.271) (36.2028, 16.477) (35.5889, 15.9905) knots 0 0 0 0 1 1 1 1
  arc A68 (37.999, 18.5031) -> (37.3046, 19.866) centre (0, 0) ccw
  spline S67 degree 3 poles (33.8552, 19.3931) (34.6096, 19.6037) (35.7503, 19.823) (37.3046, 19.866) knots 0 0 0 0 1 1 1 1
  spline S68 degree 3 poles (32.9586, 19.0846) (33.1422, 19.1638) (33.4362, 19.2759) (33.8552, 19.3931) knots 0 0 0 0 1 1 1 1
  arc A69 (32.4562, 19.2479) -> (32.9586, 19.0846) centre (32.8002, 19.4519) ccw
  arc A70 (32.4562, 19.2479) -> (31.8848, 20.1803) centre (0, 0) ccw
  arc A71 (31.9674, 20.7021) -> (31.8848, 20.1803) centre (32.2228, 20.3942) ccw
  spline S69 degree 3 poles (32.6493, 21.3609) (32.3546, 21.0408) (32.1213, 20.8297) (31.9674, 20.7021) knots 0 0 0 0 1 1 1 1
  spline S70 degree 3 poles (34.6367, 24.2197) (33.8927, 22.8543) (33.1795, 21.9375) (32.6493, 21.3609) knots 0 0 0 0 1 1 1 1
  arc A72 (34.6367, 24.2197) -> (33.7376, 25.4571) centre (0, 0) ccw
  spline S71 degree 3 poles (30.4047, 24.4505) (31.1168, 24.7765) (32.2092, 25.1715) (33.7376, 25.4571) knots 0 0 0 0 1 1 1 1
  spline S72 degree 3 poles (29.5673, 24.0055) (29.7363, 24.1124) (30.0091, 24.2691) (30.4047, 24.4505) knots 0 0 0 0 1 1 1 1
  arc A73 (29.0455, 24.0882) -> (29.5673, 24.0055) centre (29.3534, 24.3435) ccw
  arc A74 (29.0455, 24.0882) -> (28.3353, 24.9197) centre (0, 0) ccw
  arc A75 (28.3353, 25.448) -> (28.3353, 24.9197) centre (28.6357, 25.1839) ccw
  spline S73 degree 3 poles (28.9058, 26.2054) (28.6648, 25.8431) (28.4673, 25.5981) (28.3353, 25.448) knots 0 0 0 0 1 1 1 1
  spline S74 degree 3 poles (30.4214, 29.3399) (29.9002, 27.8749) (29.3392, 26.8578) (28.9058, 26.2054) knots 0 0 0 0 1 1 1 1
  arc A76 (30.4214, 29.3399) -> (29.3399, 30.4214) centre (0, 0) ccw
  spline S75 degree 3 poles (26.2054, 28.9058) (26.8578, 29.3392) (27.8749, 29.9002) (29.3399, 30.4214) knots 0 0 0 0 1 1 1 1
  spline S76 degree 3 poles (25.448, 28.3353) (25.5981, 28.4673) (25.8431, 28.6648) (26.2054, 28.9058) knots 0 0 0 0 1 1 1 1
  arc A77 (24.9197, 28.3353) -> (25.448, 28.3353) centre (25.1839, 28.6357) ccw
  arc A78 (24.9197, 28.3353) -> (24.0882, 29.0455) centre (0, 0) ccw
  arc A79 (24.0055, 29.5673) -> (24.0882, 29.0455) centre (24.3435, 29.3534) ccw
  spline S77 degree 3 poles (24.4505, 30.4047) (24.2691, 30.0091) (24.1124, 29.7363) (24.0055, 29.5673) knots 0 0 0 0 1 1 1 1
  spline S78 degree 3 poles (25.4571, 33.7376) (25.1715, 32.2092) (24.7765, 31.1168) (24.4505, 30.4047) knots 0 0 0 0 1 1 1 1
  arc A80 (25.4571, 33.7376) -> (24.2197, 34.6367) centre (0, 0) ccw
  spline S79 degree 3 poles (21.3609, 32.6493) (21.9375, 33.1795) (22.8543, 33.8927) (24.2197, 34.6367) knots 0 0 0 0 1 1 1 1
  spline S80 degree 3 poles (20.7021, 31.9674) (20.8297, 32.1213) (21.0408, 32.3546) (21.3609, 32.6493) knots 0 0 0 0 1 1 1 1
  arc A81 (20.1803, 31.8848) -> (20.7021, 31.9674) centre (20.3942, 32.2228) ccw
  arc A82 (20.1803, 31.8848) -> (19.2479, 32.4562) centre (0, 0) ccw
  arc A83 (19.0846, 32.9586) -> (19.2479, 32.4562) centre (19.4519, 32.8002) ccw
  spline S81 degree 3 poles (19.3931, 33.8552) (19.2759, 33.4362) (19.1638, 33.1422) (19.0846, 32.9586) knots 0 0 0 0 1 1 1 1
  spline S82 degree 3 poles (19.866, 37.3046) (19.823, 35.7503) (19.6037, 34.6096) (19.3931, 33.8552) knots 0 0 0 0 1 1 1 1
  arc A84 (19.866, 37.3046) -> (18.5031, 37.999) centre (0, 0) ccw
  spline S83 degree 3 poles (15.9905, 35.5889) (16.477, 36.2028) (17.271, 37.0506) (18.5031, 37.999) knots 0 0 0 0 1 1 1 1
  spline S84 degree 3 poles (15.4464, 34.8123) (15.5484, 34.9843) (15.7204, 35.2478) (15.9905, 35.5889) knots 0 0 0 0 1 1 1 1
  arc A85 (14.944, 34.6491) -> (15.4464, 34.8123) centre (15.1024, 35.0164) ccw
  arc A86 (14.944, 34.6491) -> (13.9336, 35.0676) centre (0, 0) ccw
  arc A87 (13.6938, 35.5383) -> (13.9336, 35.0676) centre (14.0813, 35.4393) ccw
  spline S85 degree 3 poles (13.8582, 36.4722) (13.808, 36.0399) (13.7432, 35.732) (13.6938, 35.5383) knots 0 0 0 0 1 1 1 1
  spline S86 degree 3 poles (13.7857, 39.953) (13.9863, 38.4112) (13.9482, 37.2502) (13.8582, 36.4722) knots 0 0 0 0 1 1 1 1
  arc A88 (13.7857, 39.953) -> (12.331, 40.4257) centre (0, 0) ccw
  spline S87 degree 3 poles (10.2263, 37.6523) (10.6107, 38.3346) (11.2623, 39.2962) (12.331, 40.4257) knots 0 0 0 0 1 1 1 1
  spline S88 degree 3 poles (9.8104, 36.8001) (9.8842, 36.9859) (10.0128, 37.273) (10.2263, 37.6523) knots 0 0 0 0 1 1 1 1
  arc A89 (9.3397, 36.5603) -> (9.8104, 36.8001) centre (9.4387, 36.9478) ccw
  arc A90 (9.3397, 36.5603) -> (8.2763, 36.8156) centre (0, 0) ccw
  arc A91 (7.9658, 37.243) -> (8.2763, 36.8156) centre (8.364, 37.2058) ccw
  spline S89 degree 3 poles (7.9821, 38.191) (8.0001, 37.7562) (7.9843, 37.442) (7.9658, 37.243) knots 0 0 0 0 1 1 1 1
  spline S90 degree 3 poles (7.3659, 41.6177) (7.8053, 40.1262) (7.9493, 38.9736) (7.9821, 38.191) knots 0 0 0 0 1 1 1 1
  arc A92 (7.3659, 41.6177) -> (5.8552, 41.857) centre (0, 0) ccw
  spline S91 degree 3 poles (4.2102, 38.7884) (4.4833, 39.5225) (4.9764, 40.5743) (5.8552, 41.857) knots 0 0 0 0 1 1 1 1
  spline S92 degree 3 poles (3.9328, 37.8817) (3.9767, 38.0767) (4.0588, 38.3805) (4.2102, 38.7884) knots 0 0 0 0 1 1 1 1
  arc A93 (3.5054, 37.5712) -> (3.9328, 37.8817) centre (3.5426, 37.9695) ccw
  arc A94 (3.5054, 37.5712) -> (2.4152, 37.657) centre (0, 0) ccw
  arc A95 (2.0416, 38.0306) -> (2.4152, 37.657) centre (2.4408, 38.0562) ccw
  spline S93 degree 3 poles (1.9094, 38.9695) (1.9952, 38.5429) (2.0288, 38.23) (2.0416, 38.0306) knots 0 0 0 0 1 1 1 1
  spline S94 degree 3 poles (0.7648, 42.2576) (1.4321, 40.8532) (1.7546, 39.7373) (1.9094, 38.9695) knots 0 0 0 0 1 1 1 1
  arc A96 (0.7648, 42.2576) -> (-0.7648, 42.2576) centre (0, 0) ccw
  spline S95 degree 3 poles (-1.9094, 38.9695) (-1.7546, 39.7373) (-1.4321, 40.8532) (-0.7648, 42.2576) knots 0 0 0 0 1 1 1 1
  spline S96 degree 3 poles (-2.0416, 38.0306) (-2.0288, 38.23) (-1.9952, 38.5429) (-1.9094, 38.9695) knots 0 0 0 0 1 1 1 1
  arc A97 (-2.4152, 37.657) -> (-2.0416, 38.0306) centre (-2.4408, 38.0562) ccw
  arc A98 (-2.4152, 37.657) -> (-3.5054, 37.5712) centre (0, 0) ccw
  arc A99 (-3.9328, 37.8817) -> (-3.5054, 37.5712) centre (-3.5426, 37.9695) ccw
  spline S97 degree 3 poles (-4.2102, 38.7884) (-4.0588, 38.3805) (-3.9767, 38.0767) (-3.9328, 37.8817) knots 0 0 0 0 1 1 1 1
  spline S98 degree 3 poles (-5.8552, 41.857) (-4.9764, 40.5743) (-4.4833, 39.5225) (-4.2102, 38.7884) knots 0 0 0 0 1 1 1 1
  arc A100 (-5.8552, 41.857) -> (-7.3659, 41.6177) centre (0, 0) ccw
  spline S99 degree 3 poles (-7.9821, 38.191) (-7.9493, 38.9736) (-7.8053, 40.1262) (-7.3659, 41.6177) knots 0 0 0 0 1 1 1 1
  spline S100 degree 3 poles (-7.9658, 37.243) (-7.9843, 37.442) (-8.0001, 37.7562) (-7.9821, 38.191) knots 0 0 0 0 1 1 1 1
  arc A101 (-8.2763, 36.8156) -> (-7.9658, 37.243) centre (-8.364, 37.2058) ccw
  arc A102 (-8.2763, 36.8156) -> (-9.3397, 36.5603) centre (0, 0) ccw
  arc A103 (-9.8104, 36.8001) -> (-9.3397, 36.5603) centre (-9.4387, 36.9478) ccw
  spline S101 degree 3 poles (-10.2263, 37.6523) (-10.0128, 37.273) (-9.8842, 36.9859) (-9.8104, 36.8001) knots 0 0 0 0 1 1 1 1
  spline S102 degree 3 poles (-12.331, 40.4257) (-11.2623, 39.2962) (-10.6107, 38.3346) (-10.2263, 37.6523) knots 0 0 0 0 1 1 1 1
  arc A104 (-12.331, 40.4257) -> (-13.7857, 39.953) centre (0, 0) ccw
  spline S103 degree 3 poles (-13.8582, 36.4722) (-13.9482, 37.2502) (-13.9863, 38.4112) (-13.7857, 39.953) knots 0 0 0 0 1 1 1 1
  spline S104 degree 3 poles (-13.6938, 35.5383) (-13.7432, 35.732) (-13.808, 36.0399) (-13.8582, 36.4722) knots 0 0 0 0 1 1 1 1
  arc A105 (-13.9336, 35.0676) -> (-13.6938, 35.5383) centre (-14.0813, 35.4393) ccw
  arc A106 (-13.9336, 35.0676) -> (-14.944, 34.6491) centre (0, 0) ccw
  arc A107 (-15.4464, 34.8123) -> (-14.944, 34.6491) centre (-15.1024, 35.0164) ccw
  spline S105 degree 3 poles (-15.9905, 35.5889) (-15.7204, 35.2478) (-15.5484, 34.9843) (-15.4464, 34.8123) knots 0 0 0 0 1 1 1 1
  spline S106 degree 3 poles (-18.5031, 37.999) (-17.271, 37.0506) (-16.477, 36.2028) (-15.9905, 35.5889) knots 0 0 0 0 1 1 1 1
  arc A108 (-18.5031, 37.999) -> (-19.866, 37.3046) centre (0, 0) ccw
  spline S107 degree 3 poles (-19.3931, 33.8552) (-19.6037, 34.6096) (-19.823, 35.7503) (-19.866, 37.3046) knots 0 0 0 0 1 1 1 1
  spline S108 degree 3 poles (-19.0846, 32.9586) (-19.1638, 33.1422) (-19.2759, 33.4362) (-19.3931, 33.8552) knots 0 0 0 0 1 1 1 1
  arc A109 (-19.2479, 32.4562) -> (-19.0846, 32.9586) centre (-19.4519, 32.8002) ccw
  arc A110 (-19.2479, 32.4562) -> (-20.1803, 31.8848) centre (0, 0) ccw
  arc A111 (-20.7021, 31.9674) -> (-20.1803, 31.8848) centre (-20.3942, 32.2228) ccw
  spline S109 degree 3 poles (-21.3609, 32.6493) (-21.0408, 32.3546) (-20.8297, 32.1213) (-20.7021, 31.9674) knots 0 0 0 0 1 1 1 1
  spline S110 degree 3 poles (-24.2197, 34.6367) (-22.8543, 33.8927) (-21.9375, 33.1795) (-21.3609, 32.6493) knots 0 0 0 0 1 1 1 1
  arc A112 (-24.2197, 34.6367) -> (-25.4571, 33.7376) centre (0, 0) ccw
  spline S111 degree 3 poles (-24.4505, 30.4047) (-24.7765, 31.1168) (-25.1715, 32.2092) (-25.4571, 33.7376) knots 0 0 0 0 1 1 1 1
  spline S112 degree 3 poles (-24.0055, 29.5673) (-24.1124, 29.7363) (-24.2691, 30.0091) (-24.4505, 30.4047) knots 0 0 0 0 1 1 1 1
  arc A113 (-24.0882, 29.0455) -> (-24.0055, 29.5673) centre (-24.3435, 29.3534) ccw
  arc A114 (-24.0882, 29.0455) -> (-24.9197, 28.3353) centre (0, 0) ccw
  arc A115 (-25.448, 28.3353) -> (-24.9197, 28.3353) centre (-25.1839, 28.6357) ccw
  spline S113 degree 3 poles (-26.2054, 28.9058) (-25.8431, 28.6648) (-25.5981, 28.4673) (-25.448, 28.3353) knots 0 0 0 0 1 1 1 1
  spline S114 degree 3 poles (-29.3399, 30.4214) (-27.8749, 29.9002) (-26.8578, 29.3392) (-26.2054, 28.9058) knots 0 0 0 0 1 1 1 1
  arc A116 (-29.3399, 30.4214) -> (-30.4214, 29.3399) centre (0, 0) ccw
  spline S115 degree 3 poles (-28.9058, 26.2054) (-29.3392, 26.8578) (-29.9002, 27.8749) (-30.4214, 29.3399) knots 0 0 0 0 1 1 1 1
  spline S116 degree 3 poles (-28.3353, 25.448) (-28.4673, 25.5981) (-28.6648, 25.8431) (-28.9058, 26.2054) knots 0 0 0 0 1 1 1 1
  arc A117 (-28.3353, 24.9197) -> (-28.3353, 25.448) centre (-28.6357, 25.1839) ccw
  arc A118 (-28.3353, 24.9197) -> (-29.0455, 24.0882) centre (0, 0) ccw
  arc A119 (-29.5673, 24.0055) -> (-29.0455, 24.0882) centre (-29.3534, 24.3435) ccw
  spline S117 degree 3 poles (-30.4047, 24.4505) (-30.0091, 24.2691) (-29.7363, 24.1124) (-29.5673, 24.0055) knots 0 0 0 0 1 1 1 1
  spline S118 degree 3 poles (-33.7376, 25.4571) (-32.2092, 25.1715) (-31.1168, 24.7765) (-30.4047, 24.4505) knots 0 0 0 0 1 1 1 1
  arc A120 (-33.7376, 25.4571) -> (-34.6367, 24.2197) centre (0, 0) ccw
  spline S119 degree 3 poles (-32.6493, 21.3609) (-33.1795, 21.9375) (-33.8927, 22.8543) (-34.6367, 24.2197) knots 0 0 0 0 1 1 1 1
  spline S120 degree 3 poles (-31.9674, 20.7021) (-32.1213, 20.8297) (-32.3546, 21.0408) (-32.6493, 21.3609) knots 0 0 0 0 1 1 1 1
  arc A121 (-31.8848, 20.1803) -> (-31.9674, 20.7021) centre (-32.2228, 20.3942) ccw
  arc A122 (-31.8848, 20.1803) -> (-32.4562, 19.2479) centre (0, 0) ccw
  arc A123 (-32.9586, 19.0846) -> (-32.4562, 19.2479) centre (-32.8002, 19.4519) ccw
  spline S121 degree 3 poles (-33.8552, 19.3931) (-33.4362, 19.2759) (-33.1422, 19.1638) (-32.9586, 19.0846) knots 0 0 0 0 1 1 1 1
  spline S122 degree 3 poles (-37.3046, 19.866) (-35.7503, 19.823) (-34.6096, 19.6037) (-33.8552, 19.3931) knots 0 0 0 0 1 1 1 1
  arc A124 (-37.3046, 19.866) -> (-37.999, 18.5031) centre (0, 0) ccw
  spline S123 degree 3 poles (-35.5889, 15.9905) (-36.2028, 16.477) (-37.0506, 17.271) (-37.999, 18.5031) knots 0 0 0 0 1 1 1 1
  spline S124 degree 3 poles (-34.8123, 15.4464) (-34.9843, 15.5484) (-35.2478, 15.7204) (-35.5889, 15.9905) knots 0 0 0 0 1 1 1 1
  arc A125 (-34.6491, 14.944) -> (-34.8123, 15.4464) centre (-35.0164, 15.1024) ccw
  arc A126 (-34.6491, 14.944) -> (-35.0676, 13.9336) centre (0, 0) ccw
  arc A127 (-35.5383, 13.6938) -> (-35.0676, 13.9336) centre (-35.4393, 14.0813) ccw
  spline S125 degree 3 poles (-36.4722, 13.8582) (-36.0399, 13.808) (-35.732, 13.7432) (-35.5383, 13.6938) knots 0 0 0 0 1 1 1 1
  spline S126 degree 3 poles (-39.953, 13.7857) (-38.4112, 13.9863) (-37.2502, 13.9482) (-36.4722, 13.8582) knots 0 0 0 0 1 1 1 1
  arc A128 (-39.953, 13.7857) -> (-40.4257, 12.331) centre (0, 0) ccw
  spline S127 degree 3 poles (-37.6523, 10.2263) (-38.3346, 10.6107) (-39.2962, 11.2623) (-40.4257, 12.331) knots 0 0 0 0 1 1 1 1
  spline S128 degree 3 poles (-36.8001, 9.8104) (-36.9859, 9.8842) (-37.273, 10.0128) (-37.6523, 10.2263) knots 0 0 0 0 1 1 1 1
  arc A129 (-36.5603, 9.3397) -> (-36.8001, 9.8104) centre (-36.9478, 9.4387) ccw
  arc A130 (-36.5603, 9.3397) -> (-36.8156, 8.2763) centre (0, 0) ccw